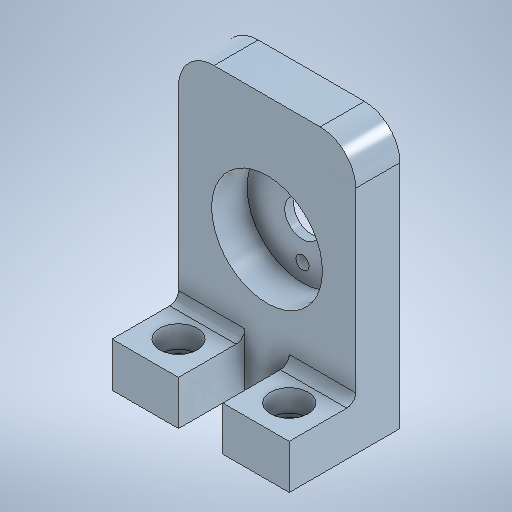
# Autodesk Inventor part: sujeción motor-acople
Saved by Autodesk Inventor 2026 (Build 300175050, 175E)
## iProperties
Created: 2025-08-26
Part Number: sujeción motor-acople
Material: Genérico
Document SubType Name: Modeling
Designer: piero
Density: 1 g/cm^3
Appearance: Valor por defecto
Author: piero
Autodesk Inventor part; units mm, degrees
ref_plane "YZ Plane" through (0, 0, 0) normal (1, 0, 0) x (0, 1, 0)
ref_plane "XZ Plane" through (0, 0, 0) normal (0, 1, 0) x (-1, 0, 0)
ref_plane "XY Plane" through (0, 0, 0) normal (0, 0, 1) x (1, 0, 0)
sketch "Boceto1" plane through (0, 0, 0) normal (0, 0, 1) x (1, 0, 0)
  line L0 (0, 0) -> (40, 0)
  line L1 (40, 0) -> (40, 60)
  line L2 (40, 60) -> (0, 60)
  line L3 (0, 60) -> (0, 0)
  circle A0 centre (20, 32) radius 4
  dimension "d0" = 40
  dimension "d1" = 60
  dimension "d2" = 8
  dimension "d31" = 32
  constraints: 8 end point, 2 parallel, 1 centre point, 1 horizontal, 1 perpendicular
  measures "d0" distance of L2.end L1.end
  measures "d1" distance of L1.end L0.end
  measures "d2" diameter of A0
  measures "d31" distance from line of A0.centre L0
extrude "Extrusión1" add sketch "Boceto1" along normal blind 10
sketch "Boceto2" plane through (0, 0, 10) normal (0, 0, 1) x (1, 0, 0)
  circle A0 centre (20, 32) radius 4 projected
  circle A1 centre (20, 32) radius 12.5
  point P0 (0, 0)
  dimension "d5" = 25
  constraints: 1 centre point, 1 coincident
  measures "d5" diameter of A1
extrude "Extrusión2" cut sketch "Boceto2" against normal blind 8
fillet "Empalme1" radius 8 2 edges at (40, 60, 5) (0, 60, 5)
sketch "Boceto4" plane through (0, 0, 0) normal (0, 0, -1) x (-1, 0, 0)
  circle A0 centre (-20, 40.5) radius 1.5
  circle A1 centre (-20, 23.5) radius 1.5
  circle A2 centre (-20, 32) radius 4 projected
  point P0 (0, 0)
  dimension "d11" = 3
  dimension "d12" = 3
  dimension "d14" = 8.5
  dimension "d15" = 17
  constraints: 2 centre point
  measures "d11" diameter of A0
  measures "d12" diameter of A1
  measures "d14" distance of A2.centre A0.centre
  measures "d15" distance of A1.centre A0.centre
extrude "Extrusión4" cut sketch "Boceto4" against normal blind 2 contours A0 | A1
sketch "Boceto5" plane through (0, 0, 10) normal (0, 0, 1) x (1, 0, 0)
  line L0 (0, 52) -> (0, 0) projected
  line L1 (0, 0) -> (15, 0)
  line L2 (15, 0) -> (15, 10)
  line L3 (15, 10) -> (0, 10)
  line L4 (0, 10) -> (0, 0)
  line L5 (40, 0) -> (40, 52) projected
  line L6 (40, 0) -> (25, 0)
  line L7 (25, 0) -> (25, 10)
  line L8 (25, 10) -> (40, 10)
  line L9 (40, 10) -> (40, 0)
  point P0 (0, 10)
  dimension "d18" = 15
  dimension "d19" = 10
  dimension "d20" = 15
  dimension "d21" = 10
  constraints: 16 end point, 4 parallel, 2 horizontal, 2 perpendicular
  measures "d18" distance of L3.end L2.end
  measures "d19" distance of L2.end L1.end
  measures "d20" distance of L7.end L8.end
  measures "d21" distance of L6.end L7.end
extrude "Extrusión5" add sketch "Boceto5" along normal blind 15
sketch "Boceto6" plane through (0, 10, 10) normal (0, 1, 0) x (1, 0, 0)
  line L0 (15, -15) -> (0, -15) projected
  line L1 (0, 0) -> (15, 0) projected
  line L2 (15, 0) -> (15, -15) projected
  circle A0 centre (7.5, -7.5) radius 3
  line L3 (25, -15) -> (40, -15) projected
  circle A1 centre (32.5, -7.5) radius 3
  circle A2 centre (7.5, -7.5) radius 4.25
  circle A3 centre (32.5, -7.5) radius 4.25
  line L4 (0, 0) -> (0, -15) projected
  line L5 (40, 0) -> (40, -15) projected
  line L6 (40, 0) -> (32, 0) projected
  point P0 (0, 10)
  point P1 (40, -7.5)
  dimension "d24" = 6
  dimension "d25" = 6
  dimension "d32" = 8.5
  dimension "d33" = 8.5
  dimension "d36" = 7.5
  dimension "d37" = 7.5
  dimension "d38" = 7.5
  dimension "d39" = 7.5
  constraints: 4 centre point, 2 coincident, 1 midpoint
  measures "d24" diameter of A0
  measures "d25" diameter of A1
  measures "d32" diameter of A2
  measures "d33" diameter of A3
  measures "d36" distance from line of A0.centre L4
  measures "d37" distance of A1.centre point (40, -7.5)
  measures "d38" distance from line of A0.centre L1
  measures "d39" distance from line of A1.centre L6
extrude "Extrusión6" cut sketch "Boceto6" against normal blind 5 contours A0 | A1
extrude "Extrusión7" cut sketch "Boceto6" against normal blind 5 contours A2 | A3
sketch "Boceto7" plane through (0, 0, 0) normal (0, -1, 0) x (1, 0, 0)
  circle A0 centre (32.5, 17.5) radius 4.25 projected
  circle A1 centre (32.5, 17.5) radius 3
  circle A2 centre (7.5, 17.5) radius 4.25 projected
  circle A3 centre (7.5, 17.5) radius 3
  point P0 (0, 0)
  dimension "d40" = 6
  dimension "d41" = 6
  constraints: 2 centre point, 2 coincident
  measures "d40" diameter of A1
  measures "d41" diameter of A3
extrude "Extrusión8" cut sketch "Boceto7" against normal blind 5 contours A1 | A3
fillet "Empalme2" radius 2 1 edges at (7.5, 10, 10)
fillet "Empalme3" radius 2 1 edges at (32.5, 10, 10)
